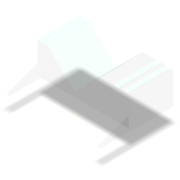
# Autodesk Inventor part: Modelo base
Saved by Autodesk Inventor 2022 (Build 260153000, 153)
## iProperties
Created: 2022-06-06
Part Number: Modelo base
Material: Generic
Document SubType Name: Modeling
Designer: ADMIN
Density: 1 g/cm^3
Appearance: Water
Author: ADMIN
Autodesk Inventor part; units mm, degrees
ref_plane "YZ Plane" through (0, 0, 0) normal (1, 0, 0) x (0, 1, 0)
ref_plane "XZ Plane" through (0, 0, 0) normal (0, 1, 0) x (-1, 0, 0)
ref_plane "XY Plane" through (0, 0, 0) normal (0, 0, 1) x (1, 0, 0)
sketch "Sketch1" plane through (0, 0, 0) normal (0, 0, 1) x (1, 0, 0)
  line L0 (-190.0993, 60.6039) -> (-190.0993, 210.6039)
  line L1 (149.9007, 210.6039) -> (149.9007, 60.6039)
  line L2 (149.9007, 60.6039) -> (-190.0993, 60.6039)
  line L3 (149.9007, 210.6039) -> (249.9007, 210.6039)
  line L4 (249.9007, 210.6039) -> (249.9007, 60.6039)
  line L5 (249.9007, 60.6039) -> (149.9007, 60.6039)
  line L6 (-190.0993, 210.6039) -> (-140.0993, 210.6039)
  line L7 (-140.0993, 210.6039) -> (-20.0993, 90.6039)
  line L8 (-20.0993, 90.6039) -> (99.9007, 210.6039)
  line L9 (99.9007, 210.6039) -> (149.9007, 210.6039)
  point P0 (0, 0)
  dimension "d0" = 340
  dimension "d1" = 150
  dimension "d2" = 150
  dimension "d3" = 170
  dimension "d5" = 100
  dimension "d16" = 90
  dimension "d17" = 50
  dimension "d18" = 50
  constraints: 20 end point, 3 perpendicular, 2 horizontal, 1 collinear, 1 parallel, 1 vertical
  measures "d0" distance of L1.end L0.start
  measures "d1" distance of L0.start L0.end
  measures "d2" distance of L1.start L1.end
  measures "d3" horizontal distance of L0.end L7.end
  measures "d5" distance of L1.start L3.end
  measures "d16" angle of L8 L7
  measures "d17" distance of L0.end L6.end
  measures "d18" distance of L8.end L1.start
extrude "Extrusion1" add sketch "Sketch1" along normal blind 200
sketch "Sketch2" plane through (0, 0, 200) normal (0, 0, 1) x (1, 0, 0)
  point P0 (0, 0)
sketch "Sketch3" plane through (249.9007, 60.6039, 0) normal (1, 0, 0) x (0, 0, -1)
  line L0 (0, 0) -> (0, 150) projected
  line L1 (0, 150) -> (-200, 150) projected
  line L2 (-200, 0) -> (-200, 150) projected
  line L3 (0, 0) -> (-200, 0) projected
  line L4 (-200, 0) -> (-350, 0)
  line L5 (-350, 0) -> (-200, 54.5955)
  line L6 (-200, 0) -> (-200, 150) projected
  point P0 (0, -60.6039)
  dimension "d12" = 20
  dimension "d13" = 150
  constraints: 4 end point, 1 horizontal, 1 point on line
  measures "d12" angle of L4 L5
  measures "d13" distance of L2.start L4.end
extrude "Extrusion2" add sketch "Sketch3" against normal blind 15 contours L4 L5 L2
sketch "Sketch4" plane through (-190.0993, 60.6039, 0) normal (-1, 0, 0) x (0, 0, 1)
  line L0 (200, 0) -> (200, 54.5955) projected
  line L1 (200, 0) -> (350, 0) projected
  line L2 (350, 0) -> (200, 54.5955) projected
  point P0 (0, -60.6039)
extrude "Extrusion3" add sketch "Sketch4" against normal blind 15
sketch "Sketch5" plane through (0, 0, 200) normal (0, 0, 1) x (1, 0, 0)
  line L0 (-119.0942, 189.5988) -> (-122.6298, 186.0633)
  line L1 (-122.6298, 186.0633) -> (-101.4166, 164.8501)
  line L2 (-101.4166, 164.8501) -> (-97.881, 168.3856)
  line L3 (-20.0993, 90.6039) -> (-140.0993, 210.6039) projected
  line L4 (-76.6678, 147.1724) -> (-80.2034, 143.6369)
  line L5 (-80.2034, 143.6369) -> (-58.9902, 122.4237)
  line L6 (-58.9902, 122.4237) -> (-55.4546, 125.9592)
  line L7 (-20.0993, 90.6039) -> (-20.0993, 149.2833) construction
  line L8 (78.8957, 189.5988) -> (82.4312, 186.0633)
  line L9 (82.4312, 186.0633) -> (61.218, 164.8501)
  line L10 (61.218, 164.8501) -> (57.6825, 168.3856)
  line L11 (36.4693, 147.1724) -> (40.0048, 143.6369)
  line L12 (40.0048, 143.6369) -> (18.7916, 122.4237)
  line L13 (18.7916, 122.4237) -> (15.256, 125.9592)
  line L14 (-175.0993, 115.1994) -> (-175.0993, 60.6039) projected
  line L15 (-175.0993, 60.6039) -> (234.9007, 60.6039) projected
  line L16 (234.9007, 60.6039) -> (234.9007, 115.1994) projected
  line L17 (234.9007, 115.1994) -> (249.9007, 115.1994) projected
  line L18 (249.9007, 115.1994) -> (249.9007, 210.6039) projected
  line L19 (249.9007, 210.6039) -> (99.9007, 210.6039) projected
  line L20 (99.9007, 210.6039) -> (-20.0993, 90.6039) projected
  line L21 (-20.0993, 90.6039) -> (-140.0993, 210.6039) projected
  line L22 (-140.0993, 210.6039) -> (-190.0993, 210.6039) projected
  line L23 (-190.0993, 210.6039) -> (-190.0993, 115.1994) projected
  line L24 (-190.0993, 115.1994) -> (-175.0993, 115.1994) projected
  line L25 (249.9007, 210.6039) -> (99.9007, 210.6039) projected
  line L26 (164.9007, 210.6039) -> (164.9007, 205.6039)
  line L27 (164.9007, 205.6039) -> (189.9007, 205.6039)
  line L28 (189.9007, 205.6039) -> (189.9007, 210.6039)
  line L29 (209.9007, 210.6039) -> (209.9007, 205.6039)
  line L30 (209.9007, 205.6039) -> (234.9007, 205.6039)
  line L31 (234.9007, 205.6039) -> (234.9007, 210.6039)
  line L32 (-140.0993, 210.6039) -> (-190.0993, 210.6039) projected
  line L33 (-177.5993, 210.6039) -> (-177.5993, 205.6039)
  line L34 (-177.5993, 205.6039) -> (-152.5993, 205.6039)
  line L35 (-152.5993, 205.6039) -> (-152.5993, 210.6039)
  point P0 (0, 0)
  point P1 (78.8957, 189.5988)
  point P2 (57.6825, 168.3856)
  point P3 (36.4693, 147.1724)
  dimension "d19" = 5
  dimension "d20" = 30
  dimension "d21" = 5
  dimension "d22" = 30
  dimension "d23" = 50
  dimension "d24" = 30
  dimension "d27" = 5
  dimension "d28" = 25
  dimension "d29" = 25
  dimension "d30" = 20
  dimension "d31" = 15
  dimension "d32" = 25
  dimension "d33" = 12.5
  dimension "d34" = 5
  constraints: 44 end point, 12 perpendicular, 10 point on line, 8 symmetric about line, 3 vertical
  measures "d19" distance of L0.start L0.end
  measures "d20" distance of L0.end L1.end
  measures "d21" distance of L4.start L4.end
  measures "d22" distance of L4.end L5.end
  measures "d23" distance from line of L3.start L6
  measures "d24" distance between parallel lines of L4 L2
  measures "d27" distance of L26.start L26.end
  measures "d28" distance of L26.end L27.end
  measures "d29" distance of L29.end L30.end
  measures "d30" distance between parallel lines of L28 L29
  measures "d31" distance between parallel lines of L18 L31
  measures "d32" distance of L33.end L34.end
  measures "d33" distance between parallel lines of L23 L33
  measures "d34" distance of L34.end L35.end
extrude "Extrusion4" cut sketch "Sketch5" against normal up to surface (200 mm away) contours L3 L2 L1 L0 | L3 L6 L5 L4 | L35 L34 L33 L22 | L20 L11 L12 L13 | L20 L8 L9 L10 | L19 L28 L27 L26 | L19 L31 L30 L29
equation "\"d2\" = d1"
equation "\"d3\" = 0.5 * d0"
equation "\"d18\" = d17"
equation "\"d21\" = d19"
equation "\"d22\" = d20"
equation "\"d27\" = d19"
equation "\"d29\" = d28"
body "Solid1"
